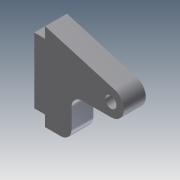
# Autodesk Inventor part: linacconnectspecial top
Saved by Autodesk Inventor 2011 (Build 150239000, 239)
## iProperties
Created: 2011-01-02
Part Number: linacconnectspecial top
Document SubType Name: Modeling
Designer: Matthew
Density: 1 g/cm^3
Author: Matthew
Autodesk Inventor part; units mm, degrees
ref_plane "YZ Plane" through (0, 0, 0) normal (1, 0, 0) x (0, 1, 0)
ref_plane "XZ Plane" through (0, 0, 0) normal (0, 1, 0) x (-1, 0, 0)
ref_plane "XY Plane" through (0, 0, 0) normal (0, 0, 1) x (1, 0, 0)
sketch "Sketch1" plane through (0, 0, 0) normal (0, 0, 1) x (1, 0, 0)
  line L0 (-23.3923, 13.9068) -> (-17.0423, 13.9068)
  line L1 (-17.0423, 13.9068) -> (-17.0423, -24.1932)
  line L2 (-17.0423, -24.1932) -> (-23.3923, -24.1932)
  line L3 (-23.3923, -24.1932) -> (-23.3923, 13.9068)
  line L4 (-17.0423, 13.9068) -> (-17.0423, 20.2568)
  line L5 (-17.0423, -24.1932) -> (-17.0423, -30.5432)
  line L6 (-17.0423, 13.9068) -> (-17.0423, 1.2068)
  line L7 (-17.0423, 1.2068) -> (21.1593, 1.2068)
  circle A0 centre (21.1593, 1.2068) radius 3.3
  line L8 (21.1593, 1.2068) -> (21.1593, -6.4132)
  line L9 (21.1593, -6.4132) -> (-1.7007, -6.4132)
  line L10 (-1.7007, -6.4132) -> (-1.7007, -30.5432)
  line L11 (-1.7007, -30.5432) -> (-17.0423, -30.5432)
  circle A1 centre (21.1593, 1.2068) radius 7.62
  line L12 (-17.0423, 20.2568) -> (23.288, 8.5234)
  point P0 (0, 0)
  dimension "d0" = 6.35
  dimension "d1" = 38.1
  dimension "d2" = 6.35
  dimension "d3" = 6.35
  dimension "d4" = 12.7
  dimension "d5" = 38.2016
  dimension "d6" = 6.6
  dimension "d7" = 7.62
  dimension "d8" = 22.86
  constraints: 26 end point, 5 perpendicular, 4 parallel, 2 centre point, 2 coincident, 2 point on circle, 1 collinear, 1 horizontal, 1 point on line, 1 tangent
  measures "d0" distance of L1.end L2.end
  measures "d1" distance of L0.end L1.end
  measures "d2" distance of L0.end L4.end
  measures "d3" distance of L1.end L5.end
  measures "d4" distance of L0.end L6.end
  measures "d5" distance of L6.end L7.end
  measures "d6" diameter of A0
  measures "d7" distance of L8.start L8.end
  measures "d8" distance of L8.end L9.end
extrude "Extrusion1" add sketch "Sketch1" along normal blind 12.7 contours L0 L1 L2 L3 | L4 L12 A1 L7 L1 | L7 A1 L9 L10 L11 L5 L1 | A1 L8 A0 L7 | L7 A0 L8 A1
fillet "Fillet1" radius 6.35 2 edges at (-1.7007, -30.5432, 6.35) (-1.7007, -6.4132, 6.35)
body "Solid1"
